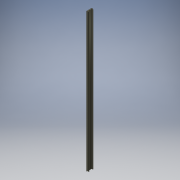
# Autodesk Inventor part: T Slot Cover 250mm
Saved by Autodesk Inventor 2016 (Build 200138000, 138)
## iProperties
Created: 2017-04-16
Part Number: T Slot Cover 250mm
Material: PC/ABS Plastic
Document SubType Name: Modeling
Designer: Scott
Density: 0.357273 g/cm^3
Appearance: Gunmetal
Author: Scott
## iProperties of the stored document T Slot Cover 250mm_3DPrint.ipt
Created: 2017-04-16
Part Number: T Slot Cover 250mm_3DPrint
Material: Generic
Document SubType Name: Modeling
Designer: Scott
Density: 1 g/cm^3
Appearance: Default
Author: Scott
Autodesk Inventor part; units mm, degrees
ref_plane "YZ Plane" through (0, 0, 0) normal (1, 0, 0) x (0, 1, 0)
ref_plane "XZ Plane" through (0, 0, 0) normal (0, 1, 0) x (-1, 0, 0)
ref_plane "XY Plane" through (0, 0, 0) normal (0, 0, 1) x (1, 0, 0)
sketch "Sketch1" plane through (0, 0, 0) normal (0, 0, 1) x (1, 0, 0)
  line L0 (0.0202, 5.1733) -> (0.0202, -4.6267)
  line L1 (0.6202, 5.1733) -> (0.6202, 4.1733)
  line L2 (1.2202, 3.2495) -> (1.2202, -2.703)
  line L3 (0.6202, 4.1733) -> (1.2202, 4.1733)
  line L4 (0.0202, 5.1733) -> (0.6202, 5.1733)
  line L5 (1.2202, 4.1733) -> (2.2202, 4.7506)
  line L6 (1.2202, 3.2495) -> (2.2202, 3.8268)
  line L7 (3.2202, 4.1733) -> (2.2202, 4.7506)
  line L8 (3.2202, 3.2495) -> (2.2202, 3.8268)
  line L9 (3.2202, 3.2495) -> (3.2202, 4.1733)
  line L10 (0.6202, -4.6267) -> (0.6202, -3.6267)
  line L11 (0.6202, -3.6267) -> (1.2202, -3.6267)
  line L12 (0.0202, -4.6267) -> (0.6202, -4.6267)
  line L13 (1.2202, -3.6267) -> (2.2202, -4.2041)
  line L14 (1.2202, -2.703) -> (2.2202, -3.2803)
  line L15 (3.2202, -3.6267) -> (2.2202, -4.2041)
  line L16 (3.2202, -2.703) -> (2.2202, -3.2803)
  line L17 (3.2202, -2.703) -> (3.2202, -3.6267)
  point P0 (0, 0)
  dimension "d0" = 120
  dimension "d1" = 120
  dimension "d2" = 90
  dimension "d3" = 60
  dimension "d4" = 2
  dimension "d5" = 2.6
  dimension "d6" = 3.2
  dimension "d7" = 0.8
  dimension "d8" = 6.955
  dimension "d9" = 7.755
  dimension "d10" = 0.8
  dimension "d11" = 6.955
  dimension "d12" = 6.155
  dimension "d13" = 7.8
  dimension "d14" = 1
  dimension "d15" = 8.8
  dimension "d16" = 3.2202
  dimension "d17" = 3.2202
  dimension "d18" = 5.2242
  dimension "d19" = 3.951
  dimension "d20" = 4.1733
  dimension "d21" = 0.6202
  constraints: 36 end point, 12 parallel, 1 horizontal, 1 vertical
  measures "d0" angle of L7 L9
  measures "d1" angle of L9 L16
  measures "d2" angle of L3 L9
  measures "d3" angle of L1 L7
  measures "d4" distance between parallel lines of L2 L17
  measures "d5" distance between parallel lines of L17 L10
  measures "d6" distance between parallel lines of L17 L0
  measures "d7" distance between parallel lines of L7 L8
  measures "d8" distance between parallel lines of L7 L14
  measures "d9" distance between parallel lines of L7 L13
  measures "d10" distance between parallel lines of L16 L15
  measures "d11" distance between parallel lines of L5 L16
  measures "d12" distance between parallel lines of L6 L16
  measures "d13" distance between parallel lines of L3 L11
  measures "d14" distance between parallel lines of L3 L4
  measures "d15" distance between parallel lines of L3 L12
  measures "d16" distance from line of point (0, 0) L9
  measures "d17" distance from line of point (0, 0) L17
  measures "d18" distance from line of point (0, 0) L7
  measures "d19" distance from line of point (0, 0) L16
  measures "d20" distance from line of point (0, 0) L3
  measures "d21" distance from line of point (0, 0) L1
extrude "Extrusion1" add sketch "Sketch1" along normal mid plane 250
body "Solid1"
